Autodesk Inventor part; units mm, degrees
(part 3 of 3)
  line L602 (884.843, 25) -> (894.843, 25)
  line L603 (589.2655, 620) -> (909.843, 620)
  line L604 (894.843, 4095) -> (889.843, 4120)
  line L605 (589.2655, 4120) -> (909.843, 4120)
  line L606 (884.843, 3795) -> (894.843, 3795)
  line L607 (894.843, 3795) -> (889.843, 3770)
  line L608 (894.843, 595) -> (889.843, 620)
  line L609 (884.843, 595) -> (889.843, 620)
  line L610 (894.843, 595) -> (884.843, 595)
  line L611 (884.843, 3795) -> (889.843, 3770)
  line L612 (589.2655, 3770) -> (909.843, 3770)
  line L613 (889.843, 3770) -> (889.843, 4120)
  line L614 (894.843, 3745) -> (884.843, 3745)
  line L615 (884.843, 3745) -> (889.843, 3770)
  line L616 (894.843, 3745) -> (889.843, 3770)
  line L617 (589.2655, 3770) -> (909.843, 3770)
  line L618 (884.843, 3445) -> (894.843, 3445)
  line L619 (894.843, 3445) -> (889.843, 3420)
  line L620 (884.843, 3445) -> (889.843, 3420)
  line L621 (589.2655, 3420) -> (909.843, 3420)
  line L622 (889.843, 3420) -> (889.843, 3770)
  line L623 (894.843, 3395) -> (884.843, 3395)
  line L624 (884.843, 3395) -> (889.843, 3420)
  line L625 (894.843, 3395) -> (889.843, 3420)
  line L626 (589.2655, 3420) -> (909.843, 3420)
  line L627 (884.843, 3095) -> (894.843, 3095)
  line L628 (894.843, 3095) -> (889.843, 3070)
  line L629 (884.843, 3095) -> (889.843, 3070)
  line L630 (589.2655, 3070) -> (909.843, 3070)
  line L631 (894.843, 4845) -> (889.843, 4820)
  line L632 (889.843, 3070) -> (889.843, 3420)
  line L633 (889.843, 0) -> (889.843, -196.0981)
  line L634 (780.4744, 0) -> (780.4744, 270)
  line L635 (639.2655, 0) -> (800.4744, 0)
  line L636 (775.4744, 25) -> (780.4744, 0)
  line L637 (785.4744, 25) -> (780.4744, 0)
  line L638 (775.4744, 25) -> (785.4744, 25)
  line L639 (589.2658, 270) -> (800.4744, 270)
  line L640 (785.4744, 245) -> (780.4744, 270)
  line L641 (775.4744, 245) -> (780.4744, 270)
  line L642 (785.4744, 245) -> (775.4744, 245)
  line L643 (780.4744, 0) -> (780.4744, -231.3398)
  line L644 (894.843, 1645) -> (884.843, 1645)
  line L645 (884.843, 1645) -> (889.843, 1670)
  line L646 (894.843, 1645) -> (889.843, 1670)
  line L647 (589.2655, 1670) -> (909.843, 1670)
  line L648 (884.843, 1345) -> (894.843, 1345)
  line L649 (894.843, 1345) -> (889.843, 1320)
  line L650 (894.843, 3045) -> (884.843, 3045)
  line L651 (884.843, 3045) -> (889.843, 3070)
  line L652 (894.843, 3045) -> (889.843, 3070)
  line L653 (884.843, 2745) -> (894.843, 2745)
  line L654 (894.843, 2745) -> (889.843, 2720)
  line L655 (884.843, 2745) -> (889.843, 2720)
  line L656 (589.2655, 2720) -> (909.843, 2720)
  line L657 (889.843, 2720) -> (889.843, 3070)
  line L658 (884.843, 1345) -> (889.843, 1320)
  line L659 (589.2655, 1320) -> (909.843, 1320)
  line L660 (889.843, 1320) -> (889.843, 1670)
  line L661 (884.843, 4845) -> (894.843, 4845)
  line L662 (589.2655, 5170) -> (909.843, 5170)
  line L663 (894.843, 5145) -> (889.843, 5170)
  line L664 (884.843, 5145) -> (889.843, 5170)
  line L665 (894.843, 5145) -> (884.843, 5145)
  line L666 (889.843, 5170) -> (889.843, 5520)
  line L667 (589.2655, 5170) -> (909.843, 5170)
  line L668 (884.843, 5195) -> (889.843, 5170)
  line L669 (894.843, 5195) -> (889.843, 5170)
  line L670 (884.843, 5195) -> (894.843, 5195)
  line L671 (589.2655, 5520) -> (621.2655, 5520)
  line L672 (656.2655, 5520) -> (909.843, 5520)
  line L673 (884.843, 4845) -> (889.843, 4820)
  line L674 (884.843, 5495) -> (889.843, 5520)
  line L675 (894.843, 5495) -> (884.843, 5495)
  line L676 (889.843, 5520) -> (889.843, 5870)
  line L677 (589.2655, 5520) -> (621.2655, 5520)
  line L678 (656.2655, 5520) -> (909.843, 5520)
  line L679 (884.843, 5545) -> (889.843, 5520)
  line L680 (894.843, 5545) -> (889.843, 5520)
  line L681 (884.843, 5545) -> (894.843, 5545)
  line L682 (589.2655, 5870) -> (909.843, 5870)
  line L683 (894.843, 5845) -> (889.843, 5870)
  line L684 (884.843, 5845) -> (889.843, 5870)
  line L685 (894.843, 5845) -> (884.843, 5845)
  line L686 (889.843, 5870) -> (889.843, 6220)
  line L687 (589.2655, 5870) -> (909.843, 5870)
  line L688 (884.843, 5895) -> (889.843, 5870)
  line L689 (894.843, 5895) -> (889.843, 5870)
  line L690 (884.843, 5895) -> (894.843, 5895)
  line L691 (589.2655, 6220) -> (909.843, 6220)
  line L692 (894.843, 6195) -> (889.843, 6220)
  line L693 (884.843, 6195) -> (889.843, 6220)
  line L694 (894.843, 6195) -> (884.843, 6195)
  line L695 (889.843, 6220) -> (889.843, 6400)
  line L696 (589.2655, 6220) -> (909.843, 6220)
  line L697 (884.843, 6245) -> (889.843, 6220)
  line L698 (894.843, 6245) -> (889.843, 6220)
  line L699 (884.843, 6245) -> (894.843, 6245)
  line L700 (629.2655, 6400) -> (909.843, 6400)
  line L701 (894.843, 6375) -> (889.843, 6400)
  line L702 (884.843, 6375) -> (889.843, 6400)
  line L703 (894.843, 6375) -> (884.843, 6375)
  line L704 (-80.7345, 6491.9106) -> (269.2658, 6491.9106)
  line L705 (-80.7345, 6410) -> (-80.7345, 6516.9106)
  line L706 (-55.7345, 6496.9106) -> (-80.7345, 6491.9106)
  line L707 (-55.7345, 6486.9106) -> (-80.7345, 6491.9106)
  line L708 (-55.7345, 6496.9106) -> (-55.7345, 6486.9106)
  line L709 (269.2658, 6349.9997) -> (269.2658, 6516.9106)
  line L710 (244.2658, 6486.9106) -> (269.2658, 6491.9106)
  line L711 (244.2658, 6496.9106) -> (269.2658, 6491.9106)
  line L712 (244.2658, 6486.9106) -> (244.2658, 6496.9106)
  line L713 (-80.7345, 6491.9106) -> (-237.9167, 6491.9106)
  line L714 (269.2658, 6491.9106) -> (619.2655, 6491.9106)
  line L715 (269.2658, 6349.9997) -> (269.2658, 6516.9106)
  line L716 (294.2658, 6496.9106) -> (269.2658, 6491.9106)
  line L717 (294.2658, 6486.9106) -> (269.2658, 6491.9106)
  line L718 (294.2658, 6496.9106) -> (294.2658, 6486.9106)
  line L719 (619.2655, 6410) -> (619.2655, 6516.9106)
  line L720 (594.2655, 6486.9106) -> (619.2655, 6491.9106)
  line L721 (594.2655, 6496.9106) -> (619.2655, 6491.9106)
  line L722 (594.2655, 6486.9106) -> (594.2655, 6496.9106)
  line L723 (708.7368, 6290) -> (708.7368, 6339.9997)
  line L724 (549.2655, 6290) -> (728.7368, 6290)
  line L725 (713.7368, 6265) -> (708.7368, 6290)
  line L726 (703.7368, 6265) -> (708.7368, 6290)
  line L727 (713.7368, 6265) -> (703.7368, 6265)
  line L728 (279.2658, 6339.9997) -> (728.7368, 6339.9997)
  line L729 (703.7368, 6364.9997) -> (708.7368, 6339.9997)
  line L730 (713.7368, 6364.9997) -> (708.7368, 6339.9997)
  line L731 (703.7368, 6364.9997) -> (713.7368, 6364.9997)
  line L732 (708.7368, 6290) -> (708.7368, 6265)
  line L733 (708.7368, 6339.9997) -> (708.7368, 6364.9997)
  line L734 (708.7368, 6339.9997) -> (708.7368, 6390)
  line L735 (279.2658, 6339.9997) -> (728.7368, 6339.9997)
  line L736 (713.7368, 6364.9997) -> (708.7368, 6339.9997)
  line L737 (703.7368, 6364.9997) -> (713.7368, 6364.9997)
  line L738 (549.2655, 6390) -> (728.7368, 6390)
  line L739 (713.7368, 6365) -> (708.7368, 6390)
  line L740 (703.7368, 6365) -> (708.7368, 6390)
  line L741 (713.7368, 6365) -> (703.7368, 6365)
  line L742 (579.2658, 340) -> (619.2655, 340)
  line L743 (579.2658, 280) -> (579.2658, 365)
  line L744 (554.2658, 335) -> (579.2658, 340)
  line L745 (554.2658, 345) -> (579.2658, 340)
  line L746 (554.2658, 335) -> (554.2658, 345)
  line L747 (619.2655, 110) -> (619.2655, 365)
  line L748 (644.2655, 345) -> (619.2655, 340)
  line L749 (644.2655, 335) -> (619.2655, 340)
  line L750 (644.2655, 345) -> (644.2655, 335)
  line L751 (579.2658, 340) -> (554.2658, 340)
  line L752 (619.2655, 340) -> (644.2655, 340)
  line L753 (589.2655, 4820) -> (909.843, 4820)
  line L754 (703.7368, 6364.9997) -> (708.7368, 6339.9997)
  line L755 (539.2655, 3940) -> (539.2655, 3840)
  line L756 (539.2655, 3840) -> (-0.7345, 3840)
  circle A71 centre (269.2655, 6340) radius 4
  line L757 (269.2655, 6332) -> (269.2655, 6348)
  line L758 (277.2655, 6340) -> (261.2655, 6340)
  line L759 (571.2655, 3770) -> (587.2655, 3770)
  line L760 (-0.7345, 6290) -> (-0.7345, 6390)
  line L761 (-0.7345, 6390) -> (539.2655, 6390)
  line L762 (539.2655, 6390) -> (539.2655, 6290)
  line L763 (539.2655, 6290) -> (-0.7345, 6290)
  line L764 (-80.7345, 6400) -> (619.2655, 6400)
  line L765 (619.2655, 6400) -> (619.2655, 6390)
  line L766 (579.2655, 6390) -> (-40.7345, 6390)
  line L767 (-80.7345, 6390) -> (-80.7345, 6400)
  line L768 (579.2655, 6390) -> (579.2655, 6400)
  line L769 (-40.7345, 6390) -> (-40.7345, 6400)
  line L770 (-0.7345, 4480) -> (-0.7345, 4580)
  line L771 (-0.7345, 4580) -> (539.2655, 4580)
  line L772 (539.2655, 4580) -> (539.2655, 4480)
  line L773 (539.2655, 4480) -> (-0.7345, 4480)
  line L774 (-0.7345, 5120) -> (-0.7345, 5220)
  line L775 (-0.7345, 5220) -> (539.2655, 5220)
  line L776 (539.2655, 5220) -> (539.2655, 5120)
  line L777 (539.2655, 5120) -> (-0.7345, 5120)
  line L778 (-0.7345, 5760) -> (-0.7345, 5860)
  line L779 (-0.7345, 5860) -> (539.2655, 5860)
  line L780 (539.2655, 5860) -> (539.2655, 5760)
  line L781 (539.2655, 5760) -> (-0.7345, 5760)
  circle A72 centre (579.2655, 620) radius 4
  line L782 (579.2655, 628) -> (579.2655, 612)
  line L783 (571.2655, 620) -> (587.2655, 620)
  circle A73 centre (579.2655, 970) radius 4
  line L784 (579.2655, 978) -> (579.2655, 962)
  line L785 (571.2655, 970) -> (587.2655, 970)
  circle A74 centre (579.2655, 1320) radius 4
  line L786 (579.2655, 1328) -> (579.2655, 1312)
  line L787 (571.2655, 1320) -> (587.2655, 1320)
  circle A75 centre (579.2655, 1670) radius 4
  line L788 (579.2655, 1678) -> (579.2655, 1662)
  line L789 (571.2655, 1670) -> (587.2655, 1670)
  circle A76 centre (579.2655, 2020) radius 4
  line L790 (579.2655, 2028) -> (579.2655, 2012)
  line L791 (571.2655, 2020) -> (587.2655, 2020)
  circle A77 centre (579.2655, 2370) radius 4
  line L792 (579.2655, 2378) -> (579.2655, 2362)
  line L793 (571.2655, 2370) -> (587.2655, 2370)
  circle A78 centre (579.2655, 2720) radius 4
  line L794 (579.2655, 2728) -> (579.2655, 2712)
  line L795 (571.2655, 2720) -> (587.2655, 2720)
  circle A79 centre (579.2655, 3070) radius 4
  line L796 (579.2655, 3078) -> (579.2655, 3062)
  line L797 (571.2655, 3070) -> (587.2655, 3070)
  circle A80 centre (579.2655, 3420) radius 4
  line L798 (579.2655, 3428) -> (579.2655, 3412)
  line L799 (571.2655, 3420) -> (587.2655, 3420)
  circle A81 centre (579.2655, 3770) radius 4
  line L800 (579.2655, 3778) -> (579.2655, 3762)
  circle A82 centre (579.2655, 4120) radius 4
  line L801 (579.2655, 4128) -> (579.2655, 4112)
  line L802 (571.2655, 4120) -> (587.2655, 4120)
  circle A83 centre (579.2655, 4470) radius 4
  line L803 (579.2655, 4478) -> (579.2655, 4462)
  line L804 (571.2655, 4470) -> (587.2655, 4470)
  circle A84 centre (579.2655, 4820) radius 4
  line L805 (579.2655, 4828) -> (579.2655, 4812)
  line L806 (571.2655, 4820) -> (587.2655, 4820)
  circle A85 centre (579.2655, 5170) radius 4
  line L807 (579.2655, 5178) -> (579.2655, 5162)
  line L808 (571.2655, 5170) -> (587.2655, 5170)
  circle A86 centre (579.2655, 5520) radius 4
  line L809 (579.2655, 5528) -> (579.2655, 5512)
  line L810 (571.2655, 5520) -> (587.2655, 5520)
  circle A87 centre (579.2655, 5870) radius 4
  line L811 (579.2655, 5878) -> (579.2655, 5862)
  line L812 (571.2655, 5870) -> (587.2655, 5870)
  circle A88 centre (579.2655, 6220) radius 4
  line L813 (579.2655, 6228) -> (579.2655, 6212)
  line L814 (571.2655, 6220) -> (587.2655, 6220)
  line L815 (-0.7345, 1280) -> (-0.7345, 1380)
  line L816 (-0.7345, 1380) -> (539.2655, 1380)
  line L817 (539.2655, 1380) -> (539.2655, 1280)
  line L818 (539.2655, 1280) -> (-0.7345, 1280)
  line L819 (-0.7345, 1920) -> (-0.7345, 2020)
  line L820 (-0.7345, 2020) -> (539.2655, 2020)
  line L821 (539.2655, 2020) -> (539.2655, 1920)
  line L822 (539.2655, 1920) -> (-0.7345, 1920)
  line L823 (-60.7345, 8) -> (-60.7345, -15)
  line L824 (-53.7345, 0) -> (-53.7345, -15)
  line L825 (-67.7345, 0) -> (-67.7345, -15)
  line L826 (599.2655, 8) -> (599.2655, -15)
  line L827 (606.2655, 0) -> (606.2655, -15)
  line L828 (592.2655, 0) -> (592.2655, -15)
  line L829 (-0.7345, 15) -> (-0.7345, -15)
  line L830 (12.2655, 0) -> (12.2655, -15)
  line L831 (-13.7345, 0) -> (-13.7345, -15)
  line L832 (539.2655, 15) -> (539.2655, -15)
  line L833 (552.2655, 0) -> (552.2655, -15)
  line L834 (526.2655, 0) -> (526.2655, -15)
  line L835 (629.2655, -15) -> (629.2655, 0)
  line L836 (629.2655, -15) -> (-90.7345, -15)
  line L837 (629.2655, 0) -> (-90.7345, 0)
  line L838 (-90.7345, 0) -> (-90.7345, -15)
  line L839 (619.2655, 0) -> (619.2655, 347.5)
  line L840 (619.2655, 382.5) -> (619.2655, 6390)
  line L841 (539.2655, 6390) -> (539.2655, 0)
  line L842 (619.2655, 6390) -> (539.2655, 6390)
  line L843 (539.2655, 3300) -> (539.2655, 3200)
  line L844 (-0.7345, 6390) -> (-80.7345, 6390)
  line L845 (-80.7345, 6390) -> (-80.7345, 0)
  line L846 (-0.7345, 0) -> (-0.7345, 6390)
  line L847 (-0.7345, 640) -> (-0.7345, 740)
  line L848 (-0.7345, 740) -> (539.2655, 740)
  line L849 (539.2655, 740) -> (539.2655, 640)
  line L850 (539.2655, 640) -> (-0.7345, 640)
  line L851 (289.2655, 100) -> (539.2655, 100)
  line L852 (539.2655, 100) -> (539.2655, 0)
  line L853 (-0.7345, 0) -> (-0.7345, 100)
  line L854 (-0.7345, 100) -> (249.2655, 100)
  line L855 (249.2655, 100) -> (269.2655, 80)
  line L856 (269.2655, 80) -> (289.2655, 100)
  circle A89 centre (579.2655, 270) radius 9
  line L857 (579.2655, 288) -> (579.2655, 252)
  line L858 (561.2655, 270) -> (597.2655, 270)
  line L859 (-0.7345, 2560) -> (-0.7345, 2660)
  line L860 (-0.7345, 2660) -> (539.2655, 2660)
  line L861 (539.2655, 2660) -> (539.2655, 2560)
  line L862 (539.2655, 2560) -> (-0.7345, 2560)
  line L863 (-0.7345, 3200) -> (-0.7345, 3300)
  line L864 (-0.7345, 3300) -> (539.2655, 3300)
  line L865 (539.2655, 3200) -> (-0.7345, 3200)
  line L866 (-0.7345, 3840) -> (-0.7345, 3940)
  line L867 (-0.7345, 3940) -> (539.2655, 3940)
  line L868 (611.2655, 5860) -> (611.2655, 5760)
  line L869 (619.2655, 5860) -> (611.2655, 5860)
  line L870 (619.2655, 5760) -> (619.2655, 5860)
  line L871 (611.2655, 5760) -> (619.2655, 5760)
  line L872 (-72.7345, 5120) -> (-72.7345, 5220)
  line L873 (-80.7345, 5120) -> (-72.7345, 5120)
  line L874 (-80.7345, 5220) -> (-80.7345, 5120)
  line L875 (-72.7345, 5220) -> (-80.7345, 5220)
  line L876 (611.2655, 5220) -> (611.2655, 5120)
  line L877 (619.2655, 5220) -> (611.2655, 5220)
  line L878 (619.2655, 5120) -> (619.2655, 5220)
  line L879 (611.2655, 5120) -> (619.2655, 5120)
  line L880 (-72.7345, 4480) -> (-72.7345, 4580)
  line L881 (-80.7345, 4480) -> (-72.7345, 4480)
  line L882 (-80.7345, 4580) -> (-80.7345, 4480)
  line L883 (-72.7345, 4580) -> (-80.7345, 4580)
  line L884 (611.2655, 4580) -> (611.2655, 4480)
  line L885 (619.2655, 4580) -> (611.2655, 4580)
  line L886 (619.2655, 4480) -> (619.2655, 4580)
  line L887 (611.2655, 4480) -> (619.2655, 4480)
  line L888 (-40.7345, 6390) -> (-80.7345, 6390)
  line L889 (619.2655, 6390) -> (579.2655, 6390)
  line L890 (-72.7345, 6290) -> (-72.7345, 6390)
  line L891 (-80.7345, 6290) -> (-72.7345, 6290)
  line L892 (-80.7345, 6390) -> (-80.7345, 6290)
  line L893 (-72.7345, 6390) -> (-80.7345, 6390)
  line L894 (611.2655, 6390) -> (611.2655, 6290)
  line L895 (619.2655, 6390) -> (611.2655, 6390)
  line L896 (619.2655, 6290) -> (619.2655, 6390)
  line L897 (-80.7345, 5860) -> (-80.7345, 5760)
  line L898 (611.2655, 100) -> (611.2655, 0)
  line L899 (619.2655, 100) -> (611.2655, 100)
  line L900 (619.2655, 0) -> (619.2655, 100)
  line L901 (611.2655, 0) -> (619.2655, 0)
  line L902 (539.2655, 0) -> (-0.7345, 0)
  line L903 (611.2655, 740) -> (611.2655, 640)
  line L904 (619.2655, 740) -> (611.2655, 740)
  line L905 (619.2655, 640) -> (619.2655, 740)
  line L906 (611.2655, 640) -> (619.2655, 640)
  line L907 (-72.7345, 0) -> (-72.7345, 100)
  line L908 (-80.7345, 0) -> (-72.7345, 0)
  line L909 (-80.7345, 100) -> (-80.7345, 0)
  line L910 (-72.7345, 100) -> (-80.7345, 100)
  line L911 (-72.7345, 640) -> (-72.7345, 740)
  line L912 (-80.7345, 640) -> (-72.7345, 640)
  line L913 (-80.7345, 740) -> (-80.7345, 640)
  line L914 (-72.7345, 740) -> (-80.7345, 740)
  line L915 (-72.7345, 0) -> (-72.7345, 6390)
  line L916 (-80.7345, 0) -> (-0.7345, 0)
  line L917 (611.2655, 347.5) -> (611.2655, 0)
  line L918 (611.2655, 6390) -> (611.2655, 382.5)
  line L919 (539.2655, 0) -> (619.2655, 0)
  line L920 (611.2655, 6290) -> (619.2655, 6290)
  line L921 (-72.7345, 1920) -> (-72.7345, 2020)
  line L922 (-80.7345, 1920) -> (-72.7345, 1920)
  line L923 (-80.7345, 2020) -> (-80.7345, 1920)
  line L924 (-72.7345, 2020) -> (-80.7345, 2020)
  line L925 (611.2655, 2020) -> (611.2655, 1920)
  line L926 (619.2655, 2020) -> (611.2655, 2020)
  line L927 (619.2655, 1920) -> (619.2655, 2020)
  line L928 (611.2655, 1920) -> (619.2655, 1920)
  line L929 (-72.7345, 1280) -> (-72.7345, 1380)
  line L930 (-80.7345, 1280) -> (-72.7345, 1280)
  line L931 (-80.7345, 1380) -> (-80.7345, 1280)
  line L932 (-72.7345, 1380) -> (-80.7345, 1380)
  line L933 (611.2655, 1380) -> (611.2655, 1280)
  line L934 (619.2655, 1380) -> (611.2655, 1380)
  line L935 (619.2655, 1280) -> (619.2655, 1380)
  line L936 (611.2655, 1280) -> (619.2655, 1280)
  line L937 (-72.7345, 5760) -> (-72.7345, 5860)
  line L938 (-72.7345, 3840) -> (-72.7345, 3940)
  line L939 (-80.7345, 3840) -> (-72.7345, 3840)
  line L940 (-80.7345, 3940) -> (-80.7345, 3840)
  line L941 (-72.7345, 3940) -> (-80.7345, 3940)
  line L942 (611.2655, 3940) -> (611.2655, 3840)
  line L943 (619.2655, 3940) -> (611.2655, 3940)
  line L944 (619.2655, 3840) -> (619.2655, 3940)
  line L945 (611.2655, 3840) -> (619.2655, 3840)
  line L946 (-72.7345, 3200) -> (-72.7345, 3300)
  line L947 (-80.7345, 3200) -> (-72.7345, 3200)
  line L948 (-80.7345, 3300) -> (-80.7345, 3200)
  line L949 (-72.7345, 3300) -> (-80.7345, 3300)
  line L950 (611.2655, 3300) -> (611.2655, 3200)
  line L951 (619.2655, 3300) -> (611.2655, 3300)
  line L952 (619.2655, 3200) -> (619.2655, 3300)
  line L953 (611.2655, 3200) -> (619.2655, 3200)
  line L954 (-72.7345, 2560) -> (-72.7345, 2660)
  line L955 (-80.7345, 2560) -> (-72.7345, 2560)
  line L956 (-80.7345, 2660) -> (-80.7345, 2560)
  line L957 (-72.7345, 2660) -> (-80.7345, 2660)
  line L958 (611.2655, 2660) -> (611.2655, 2560)
  line L959 (619.2655, 2660) -> (611.2655, 2660)
  line L960 (619.2655, 2560) -> (619.2655, 2660)
  line L961 (611.2655, 2560) -> (619.2655, 2560)
  line L962 (-80.7345, 5760) -> (-72.7345, 5760)
  line L963 (-72.7345, 5860) -> (-80.7345, 5860)
  line L964 (333.6357, 347.7871) -> (455.2646, 347.7871)
  line L965 (333.6357, 384.7871) -> (455.2646, 384.7871)
  line L966 (455.2646, 347.7871) -> (455.2646, 384.7871)
  line L967 (333.6357, 347.7871) -> (333.6357, 384.7871)
  line L968 (579.2652, 269.9997) -> (485.2646, 372.4538)
  line L969 (485.2646, 372.4538) -> (455.2646, 372.4538)
  line L970 (-210.274, 0) -> (-199.7739, 35)
  line L971 (722.9847, 100) -> (722.9847, 0)
  line L972 (733.4849, 35) -> (712.4849, 35)
  line L973 (745.7347, -0.0001) -> (687.9847, 0.0001)
  line L974 (722.9847, 0) -> (712.4849, 35)
  line L975 (722.9847, 0) -> (733.4849, 35)
  line L976 (-210.274, 100) -> (-210.274, 0)
  line L977 (-210.274, 0) -> (-220.7739, 35)
  line L978 (340.3265, 6229.1613) -> (446.9529, 6229.1613)
  line L979 (340.3265, 6266.1613) -> (446.9529, 6266.1613)
  line L980 (446.9529, 6229.1613) -> (446.9529, 6266.1613)
  line L981 (340.3265, 6229.1613) -> (340.3265, 6266.1613)
  line L982 (270.5015, 6343.8042) -> (310.3265, 6253.8279)
  line L983 (310.3265, 6253.8279) -> (340.3265, 6253.8279)
  line L984 (-199.7739, 35) -> (-220.7739, 35)
  line L985 (272.4809, 535.8236) -> (468.5483, 535.8236)
  line L986 (272.4809, 572.8236) -> (468.5483, 572.8236)
  line L987 (468.5483, 535.8236) -> (468.5483, 572.8236)
  line L988 (272.4809, 535.8236) -> (272.4809, 572.8236)
  line L989 (579.2655, 620) -> (498.5483, 560.4903)
  line L990 (498.5483, 560.4903) -> (468.5483, 560.4903)
  line L991 (-175.274, -0.0001) -> (-233.024, 0.0001)
  line L992 (94.1194, 6604.5956) -> (449.8616, 6604.5956)
  arc A90 (620.2655, 5504.9949) -> (657.2655, 5504.9949) centre (638.7655, 5504.9949) ccw
  arc A91 (657.2655, 5598.5623) -> (620.2655, 5598.5623) centre (638.7655, 5598.5623) ccw
  line L993 (620.2655, 5504.9949) -> (620.2655, 5598.5623)
  line L994 (657.2655, 5504.9949) -> (657.2655, 5598.5623)
  arc A92 (51.7655, 1418) -> (51.7655, 1381) centre (51.7655, 1399.5) ccw
  arc A93 (154.5614, 1381) -> (154.5614, 1418) centre (154.5614, 1399.5) ccw
  line L995 (51.7655, 1418) -> (154.5614, 1418)
  line L996 (51.7655, 1381) -> (154.5614, 1381)
  arc A94 (51.7655, 2058) -> (51.7655, 2021) centre (51.7655, 2039.5) ccw
  arc A95 (154.5614, 2021) -> (154.5614, 2058) centre (154.5614, 2039.5) ccw
  line L997 (51.7655, 2058) -> (154.5614, 2058)
  line L998 (51.7655, 2021) -> (154.5614, 2021)
  arc A96 (-151.2345, 5449.5275) -> (-81.7345, 5449.5275) centre (-116.4845, 5449.5275) ccw
  arc A97 (-81.7345, 5660.3899) -> (-151.2345, 5660.3899) centre (-116.4845, 5660.3899) ccw
  line L999 (-151.2345, 5449.5275) -> (-151.2345, 5660.3899)
  line L1000 (-81.7345, 5449.5275) -> (-81.7345, 5660.3899)
  arc A98 (42.4942, 138) -> (42.4942, 101) centre (42.4942, 119.5) ccw
  arc A99 (145.2901, 101) -> (145.2901, 138) centre (145.2901, 119.5) ccw
  line L1001 (42.4942, 138) -> (145.2901, 138)
  line L1002 (42.4942, 101) -> (145.2901, 101)
  arc A100 (42.4942, 778) -> (42.4942, 741) centre (42.4942, 759.5) ccw
  arc A101 (145.2901, 741) -> (145.2901, 778) centre (145.2901, 759.5) ccw
  line L1003 (42.4942, 778) -> (145.2901, 778)
  line L1004 (51.7655, 5861) -> (154.5614, 5861)
  line L1005 (51.7655, 5898) -> (154.5614, 5898)
  arc A102 (154.5614, 5861) -> (154.5614, 5898) centre (154.5614, 5879.5) ccw
  arc A103 (51.7655, 5898) -> (51.7655, 5861) centre (51.7655, 5879.5) ccw
  line L1006 (51.7655, 5221) -> (154.5614, 5221)
  line L1007 (51.7655, 5258) -> (154.5614, 5258)
  arc A104 (154.5614, 5221) -> (154.5614, 5258) centre (154.5614, 5239.5) ccw
  arc A105 (51.7655, 5258) -> (51.7655, 5221) centre (51.7655, 5239.5) ccw
  line L1008 (51.7655, 4581) -> (154.5614, 4581)
  line L1009 (51.7655, 4618) -> (154.5614, 4618)
  arc A106 (154.5614, 4581) -> (154.5614, 4618) centre (154.5614, 4599.5) ccw
  arc A107 (51.7655, 4618) -> (51.7655, 4581) centre (51.7655, 4599.5) ccw
  line L1010 (-32.2055, 6409.0391) -> (70.5904, 6409.0391)
  line L1011 (42.4942, 741) -> (145.2901, 741)
  arc A108 (70.5904, 6409.0391) -> (70.5904, 6446.0391) centre (70.5904, 6427.5391) ccw
  arc A109 (-32.2055, 6446.0391) -> (-32.2055, 6409.0391) centre (-32.2055, 6427.5391) ccw
  line L1012 (-60.4895, 6399.2551) -> (-32.2055, 6409.0391)
  line L1013 (132.5595, 6248.494) -> (235.3554, 6248.494)
  line L1014 (132.5595, 6285.494) -> (235.3554, 6285.494)
  arc A110 (235.3554, 6248.494) -> (235.3554, 6285.494) centre (235.3554, 6266.994) ccw
  arc A111 (132.5595, 6285.494) -> (132.5595, 6248.494) centre (132.5595, 6266.994) ccw
  line L1015 (107.5595, 6310.294) -> (132.5595, 6285.494)
  line L1016 (51.7655, 3941) -> (154.5614, 3941)
  line L1017 (51.7655, 3978) -> (154.5614, 3978)
  arc A112 (154.5614, 3941) -> (154.5614, 3978) centre (154.5614, 3959.5) ccw
  arc A113 (51.7655, 3978) -> (51.7655, 3941) centre (51.7655, 3959.5) ccw
  line L1018 (51.7655, 3301) -> (154.5614, 3301)
  line L1019 (51.7655, 3338) -> (154.5614, 3338)
  arc A114 (154.5614, 3301) -> (154.5614, 3338) centre (154.5614, 3319.5) ccw
  arc A115 (51.7655, 3338) -> (51.7655, 3301) centre (51.7655, 3319.5) ccw
  line L1020 (51.7655, 2661) -> (154.5614, 2661)
  line L1021 (51.7655, 2698) -> (154.5614, 2698)
  arc A116 (154.5614, 2661) -> (154.5614, 2698) centre (154.5614, 2679.5) ccw
  arc A117 (51.7655, 2698) -> (51.7655, 2661) centre (51.7655, 2679.5) ccw
  line L1022 (-32.2055, 6446.0391) -> (70.5904, 6446.0391)
  point P0 (270, -15)
  point P1 (33682.2925, 14686.87)
  point P2 (33340.0195, 14686.87)
  point P3 (33050.2135, 14867.4)
  point P4 (34040.0195, 14686.87)
  point P5 (33035.7555, 21267.4)
  point P6 (34303.0776, 17399.5863)
  point P7 (34303.0776, 19499.5863)
  point P8 (34303.0776, 15999.5863)
  point P9 (34303.0776, 19149.5863)
  point P10 (34303.0776, 18799.5863)
  point P11 (34303.0776, 17049.5863)
  point P12 (34303.0776, 15649.5863)
  point P13 (34303.0776, 16699.5863)
  point P14 (34303.0776, 15164.5863)
  point P15 (34303.0776, 18449.5863)
  point P16 (34303.0776, 14694.3019)
  point P17 (34303.0776, 18099.5863)
  point P18 (34353.0776, 14722.0729)
  point P19 (34193.709, 14989.5863)
  point P20 (34193.709, 14659.0602)
  point P21 (34243.709, 14722.0729)
  point P22 (34303.0776, 16349.5863)
  point P23 (34303.0776, 17749.5863)
  point P24 (34303.0776, 19849.5863)
  point P25 (34303.0776, 20199.5863)
  point P26 (34303.0776, 20549.5863)
  point P27 (34303.0776, 20899.5863)
  point P28 (34303.0776, 21164.5863)
  point P29 (33492.1864, 21386.8106)
  point P30 (33195.8179, 21386.8106)
  point P31 (33842.1864, 21386.8106)
  point P32 (34121.9714, 21178.8574)
  point P33 (34121.9714, 21228.8574)
  point P34 (34006.4577, 15234.9)
  point P35 (33813.0363, 15236.1871)
  point P36 (33765.3703, 15236.1871)
  point P37 (33235.4605, 14932.4)
  point P38 (33819.727, 21117.5613)
  point P39 (34089.6958, 14932.4)
  point P40 (33787.8727, 15236.1871)
  point P41 (33772.061, 21117.5613)
  point P42 (33794.5634, 21117.5613)
  point P43 (33747.067, 15424.2236)
  point P44 (33841.3224, 15424.2236)
  point P45 (33704.2155, 15424.2236)
  point P46 (33667.5675, 21454.4956)
  point P47 (33519.8539, 21494.4956)
  point P48 (34077, 20393.3949)
  point P49 (33483.5, 16269.4)
  point P50 (33483.5, 16909.4)
  point P51 (33305.5, 20436.6263)
  point P52 (33338, 20337.9275)
  point P53 (33305.5, 20455.2225)
  point P54 (33305.5, 20337.9275)
  point P55 (33474.2288, 14989.4)
  point P56 (33483.5, 20749.4)
  point P57 (33483.5, 20109.4)
  point P58 (33483.5, 19469.4)
  point P59 (33399.529, 21297.4391)
  point P60 (33564.294, 21136.894)
  point P61 (33483.5, 18829.4)
  point P62 (33483.5, 18189.4)
  point P63 (33483.5, 17549.4)
  point P64 (33474.2288, 15629.4)
  point P65 (256.5579, -195.53)
  point P66 (-85.715, -195.53)
  point P67 (-375.5211, -15)
  point P68 (614.285, -195.53)
  point P69 (-389.9791, 6385)
  point P70 (877.343, 2517.1863)
  point P71 (877.343, 4617.1863)
  point P72 (877.343, 1117.1863)
  point P73 (877.343, 4267.1863)
  point P74 (877.343, 3917.1863)
  point P75 (877.343, 2167.1863)
  point P76 (877.343, 767.1863)
  point P77 (877.343, 1817.1863)
  point P78 (877.343, 282.1863)
  point P79 (877.343, 3567.1863)
  point P80 (877.343, -188.0981)
  point P81 (877.343, 3217.1863)
  point P82 (927.343, -160.3271)
  point P83 (767.9744, 107.1863)
  point P84 (767.9744, -223.3398)
  point P85 (817.9744, -160.3271)
  point P86 (877.343, 1467.1863)
  point P87 (877.343, 2867.1863)
  point P88 (877.343, 4967.1863)
  point P89 (877.343, 5317.1863)
  point P90 (877.343, 5667.1863)
  point P91 (877.343, 6017.1863)
  point P92 (877.343, 6282.1863)
  point P93 (66.4519, 6504.4106)
  point P94 (-229.9167, 6504.4106)
  point P95 (416.4519, 6504.4106)
  point P96 (696.2368, 6296.4574)
  point P97 (696.2368, 6346.4574)
  point P98 (580.7231, 352.5)
  point P99 (387.3017, 353.7871)
  point P100 (339.6357, 353.7871)
  point P101 (-190.274, 50)
  point P102 (393.9925, 6235.1613)
  point P103 (663.9613, 50)
  point P104 (362.1382, 353.7871)
  point P105 (346.3265, 6235.1613)
  point P106 (368.8289, 6235.1613)
  point P107 (321.3325, 541.8236)
  point P108 (415.5878, 541.8236)
  point P109 (278.4809, 541.8236)
  point P110 (241.833, 6572.0956)
  point P111 (94.1194, 6612.0956)
  point P112 (651.2655, 5510.9949)
  point P113 (57.7655, 1387)
  point P114 (57.7655, 2027)
  point P115 (-120.2345, 5554.2263)
  point P116 (-87.7345, 5455.5275)
  point P117 (-120.2345, 5572.8225)
  point P118 (-120.2345, 5455.5275)
  point P119 (48.4942, 107)
  point P120 (57.7655, 5867)
  point P121 (57.7655, 5227)
  point P122 (57.7655, 4587)
  point P123 (-26.2055, 6415.0391)
  point P124 (138.5595, 6254.494)
  point P125 (57.7655, 3947)
  point P126 (57.7655, 3307)
  point P127 (57.7655, 2667)
  point P128 (48.4942, 747)
  constraints: 2000 end point, 222 point on line, 164 point on circle, 116 centre point, 26 midpoint, 630 other
sketch "Sketch9" plane through (-270, 15, 350) normal (0, 0, 1) x (1, 0, 0)
  line L0 (249.2655, 100) -> (269.2655, 80) projected
  line L1 (269.2655, 80) -> (289.2655, 100) projected
  line L2 (249.2655, 100) -> (289.2655, 100)
  line L3 (0, 100) -> (540, 100) projected
  circle A0 centre (579.2655, 270) radius 9 projected
  circle A1 centre (579.2655, 620) radius 4 projected
  circle A2 centre (579.2655, 970) radius 4 projected
  circle A3 centre (579.2655, 1320) radius 4 projected
  circle A4 centre (579.2655, 1670) radius 4 projected
  circle A5 centre (579.2655, 2020) radius 4 projected
  circle A6 centre (579.2655, 2370) radius 4 projected
  circle A7 centre (579.2655, 2720) radius 4 projected
  circle A8 centre (579.2655, 3070) radius 4 projected
  circle A9 centre (579.2655, 3420) radius 4 projected
  circle A10 centre (579.2655, 3770) radius 4 projected
  circle A11 centre (579.2655, 4120) radius 4 projected
  circle A12 centre (579.2655, 4470) radius 4 projected
  circle A13 centre (579.2655, 4820) radius 4 projected
  circle A14 centre (579.2655, 5170) radius 4 projected
  circle A15 centre (579.2655, 5520) radius 4 projected
  circle A16 centre (579.2655, 5870) radius 4 projected
  circle A17 centre (579.2655, 6220) radius 4 projected
  circle A18 centre (269.2655, 6340) radius 4 projected
  point P0 (270, -15)
  constraints: 2 end point, 1 collinear
extrude "Extrusion19" cut sketch "Sketch9" against normal blind 15 contours L2 L1 L0 bodies 6
extrude "Extrusion20" cut sketch "Sketch9" against normal blind 15 contours A0 | A1 | A2 | A3 | A4 | A5 | A6 | A7 | A8 | A9 | A10 | A11 | A12 | A13 | A14 | A15 | A16 | A17 bodies 3
extrude "Extrusion21" cut sketch "Sketch9" against normal blind 15 contours A18 bodies 16
body "Solid1"
body "Solid2"
body "Solid3"
body "Solid4"
body "Solid5"
body "Solid6"
body "Solid7"
body "Solid8"
body "Solid9"
body "Solid10"
body "Solid11"
body "Solid12"
body "Solid13"
body "Solid14"
body "Solid15"
body "Solid16"
body "Solid17"
